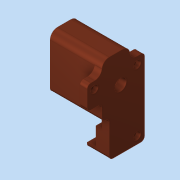
# Autodesk Inventor part: limitSwitchPushHolder1
Saved by Autodesk Inventor 2017 (Build 210142000, 142)
## iProperties
Created: 2016-12-04
Part Number: limitSwitchPushHolder1
Material: ABS Plastic
Document SubType Name: Modeling
Designer: techn
Density: 1.06 g/cm^3
Appearance: Copper - Satin
Author: techn
Autodesk Inventor part; units mm, degrees
ref_plane "YZ Plane" through (0, 0, 0) normal (1, 0, 0) x (0, 1, 0)
ref_plane "XZ Plane" through (0, 0, 0) normal (0, 1, 0) x (-1, 0, 0)
ref_plane "XY Plane" through (0, 0, 0) normal (0, 0, 1) x (1, 0, 0)
sketch "Sketch1" plane through (0, 0, 0) normal (0, 0, 1) x (1, 0, 0)
  line L0 (0, 0) -> (-2.54, 0)
  line L1 (-2.54, 0) -> (-2.54, 7.62)
  line L2 (-2.54, 7.62) -> (0, 7.62)
  line L3 (0, 7.62) -> (0, 0)
  line L4 (-2.54, 7.62) -> (18.796, 7.62)
  line L5 (18.796, 7.62) -> (18.796, 10.16)
  line L6 (18.796, 10.16) -> (-2.54, 10.16)
  line L7 (-2.54, 10.16) -> (-2.54, 7.62)
  line L8 (11.43, -20.32) -> (16.256, -20.32)
  line L9 (16.256, -20.32) -> (16.256, -22.86)
  line L10 (16.256, -22.86) -> (11.43, -22.86)
  line L11 (11.43, -22.86) -> (11.43, -20.32)
  line L12 (16.256, -22.86) -> (18.796, -22.86)
  line L13 (18.796, -22.86) -> (18.796, -12.7)
  line L14 (18.796, -12.7) -> (16.256, -12.7)
  line L15 (16.256, -12.7) -> (16.256, -22.86)
  line L16 (-2.54, 10.16) -> (18.796, 10.16)
  line L17 (18.796, 10.16) -> (18.796, -22.86)
  line L18 (18.796, -22.86) -> (-2.54, -22.86)
  line L19 (-2.54, -22.86) -> (-2.54, 10.16)
  dimension "d0" = 2.54
  dimension "d1" = 7.62
  dimension "d3" = 2.54
  dimension "d4" = 27.94
  dimension "d5" = 11.43
  dimension "d6" = 4.826
  dimension "d7" = 2.54
  dimension "d8" = 2.54
  dimension "d9" = 10.16
  constraints: 40 end point, 10 parallel, 5 horizontal, 5 perpendicular, 1 point on line
  measures "d0" distance of L1.end L2.end
  measures "d1" distance of L0.end L1.end
  measures "d3" distance of L5.end L4.end
  measures "d4" distance from line of L8.start L4
  measures "d5" horizontal distance of L2.end L8.start
  measures "d6" distance of L9.end L10.end
  measures "d7" distance of L8.end L9.end
  measures "d8" distance of L14.end L13.end
  measures "d9" distance of L13.end L12.end
extrude "Extrusion1" add sketch "Sketch1" against normal blind 8.89 contours L0 L1 L2 L3 | L2 L7 L6 L5 L4 | L11 L8 L9 L10 | L13 L12 L9 L15 L14
extrude "Extrusion2" add sketch "Sketch1" along normal blind 3.175
sketch "Sketch5" plane through (18.796, -22.86, -8.89) normal (1, 0, 0) x (0, 0, -1)
  line L0 (-8.89, 33.02) -> (-12.065, 33.02) projected
  line L1 (-12.065, 0) -> (0, 0) projected
  line L2 (0, 33.02) -> (0, 30.48) projected
  line L3 (-18.415, 33.02) -> (6.35, 33.02)
  line L4 (6.35, 33.02) -> (6.35, 0)
  line L5 (6.35, 0) -> (-18.415, 0)
  line L6 (-18.415, 0) -> (-18.415, 33.02)
  line L7 (-12.065, 0) -> (-12.065, 33.02) projected
  circle A0 centre (-15.24, 29.845) radius 1.5875
  circle A1 centre (3.175, 29.845) radius 1.5875
  circle A2 centre (-15.24, 3.175) radius 1.5875
  circle A3 centre (3.175, 3.175) radius 1.5875
  point P0 (-8.89, 22.86)
  dimension "d27" = 6.35
  dimension "d28" = 6.35
  dimension "d29" = 3.175
  dimension "d30" = 3.175
  dimension "d31" = 3.175
  dimension "d32" = 3.175
  dimension "d33" = 3.175
  dimension "d34" = 3.175
  dimension "d35" = 3.175
  dimension "d36" = 3.175
  dimension "d37" = 3.175
  dimension "d38" = 3.175
  dimension "d39" = 3.175
  dimension "d40" = 3.175
  constraints: 8 end point, 4 centre point, 2 parallel, 1 horizontal, 1 perpendicular
  measures "d27" distance between parallel lines of L7 L6
  measures "d28" distance between parallel lines of L2 L4
  measures "d29" diameter of A0
  measures "d30" diameter of A1
  measures "d31" diameter of A2
  measures "d32" diameter of A3
  measures "d33" distance from line of L7 A0.centre
  measures "d34" distance from line of A1.centre L2
  measures "d35" distance from line of L2 A3.centre
  measures "d36" distance from line of L7 A2.centre
  measures "d37" distance from line of L5 A2.centre
  measures "d38" distance from line of L3 A0.centre
  measures "d39" distance from line of L3 A1.centre
  measures "d40" distance from line of L5 A3.centre
extrude "Extrusion5" add sketch "Sketch5" along normal blind 3.175
chamfer "Chamfer2" distance 1.27 angle 45 4 edges at (18.796, 6.985, -10.4775) (18.796, -19.685, -10.4775) (18.796, -19.685, 7.9375) (18.796, 6.985, 7.9375)
sketch "Sketch7" plane through (21.971, -22.86, -8.89) normal (1, 0, 0) x (0, 0, -1)
  line L0 (-8.89, 10.16) -> (-8.89, 30.48) projected
  circle A0 centre (-4.0005, 25.908) radius 2.54
  line L1 (6.35, 33.02) -> (-18.415, 33.02) projected
  point P0 (-8.89, 22.86)
  dimension "d52" = 5.08
  dimension "d53" = 4.8895
  dimension "d54" = 7.112
  constraints: 1 centre point
  measures "d52" diameter of A0
  measures "d53" distance from line of A0.centre L0
  measures "d54" distance from line of A0.centre L1
extrude "Extrusion7" cut sketch "Sketch7" against normal blind 3.175
sketch "Sketch9" plane through (21.971, -22.86, -8.89) normal (1, 0, 0) x (0, 0, -1)
  line L0 (-18.415, 33.02) -> (-18.415, 0) projected
  line L1 (6.35, 33.02) -> (-18.415, 33.02) projected
  line L2 (-18.415, 0) -> (6.35, 0) projected
  line L3 (-18.415, 22.86) -> (-12.065, 22.86)
  line L4 (-12.065, 22.86) -> (-12.065, 0)
  line L5 (-12.065, 0) -> (-18.415, 0)
  line L6 (-18.415, 0) -> (-18.415, 22.86)
  point P0 (-8.89, 22.86)
  dimension "d59" = 6.35
  dimension "d60" = 22.86
  constraints: 8 end point, 2 parallel, 2 point on line, 1 horizontal, 1 perpendicular
  measures "d59" distance of L4.end L5.end
  measures "d60" distance of L3.end L4.end
extrude "Extrusion8" cut sketch "Sketch9" against normal through all
sketch "Sketch12" plane through (0, 0, -8.89) normal (0, 0, -1) x (-1, 0, 0)
  line L0 (-11.43, -20.32) -> (-11.43, -22.86) projected
  line L1 (2.54, -22.86) -> (-21.971, -22.86) projected
  line L2 (-11.43, -20.32) -> (-12.446, -20.32)
  line L3 (-12.446, -20.32) -> (-12.446, -22.86)
  line L4 (-12.446, -22.86) -> (-11.43, -22.86)
  line L5 (-11.43, -22.86) -> (-11.43, -20.32)
  point P0 (0, 0)
  dimension "d69" = 1.016
  constraints: 8 end point, 2 parallel, 1 horizontal, 1 perpendicular, 1 point on line
  measures "d69" distance of L4.end L3.end
extrude "Extrusion9" cut sketch "Sketch12" against normal up to surface (8.89 mm away)
sketch "Sketch16" plane through (21.971, -22.86, -8.89) normal (1, 0, 0) x (0, 0, -1)
  line L0 (-8.89, 10.16) -> (-8.89, 30.48) projected
  line L1 (-12.065, 33.02) -> (-12.065, 0) projected
  line L2 (-8.89, 22.86) -> (-8.89, 0) projected
  line L3 (-12.065, 15.875) -> (-8.89, 15.875)
  line L4 (-8.89, 15.875) -> (-8.89, 0)
  line L5 (-8.89, 0) -> (-12.065, 0)
  line L6 (-12.065, 0) -> (-12.065, 15.875)
  dimension "d74" = 15.875
  constraints: 8 end point, 2 parallel, 1 horizontal, 1 perpendicular, 1 point on line
  measures "d74" distance between parallel lines of L5 L3
extrude "Extrusion10" cut sketch "Sketch16" against normal through all
fillet "Fillet1" radius 1.5875 2 edges at (9.7155, -6.985, 3.175) (20.3835, -6.985, 0)
fillet "Fillet2" radius 1.5875 6 edges at (20.3835, 0, 9.525) (20.3835, 0, 3.175) (17.2085, -22.86, 0) (20.3835, -22.86, -15.24) (20.3835, 10.16, -15.24) (20.3835, 10.16, 9.525)
sketch "Sketch17" plane through (-2.54, 0, -8.89) normal (-1, 0, 0) x (0, 0, 1)
  arc A0 (10.4775, -6.985) -> (12.065, -5.3975) centre (10.4775, -5.3975) ccw projected
  line L0 (12.065, 10.16) -> (12.065, -5.3975) projected
  line L1 (0, 10.16) -> (12.065, 10.16) projected
  line L2 (0, 0) -> (0, 10.16) projected
  line L3 (8.89, 0) -> (0, 0) projected
  line L4 (8.89, 0) -> (8.89, -6.985) projected
  line L5 (8.89, -6.985) -> (10.4775, -6.985) projected
  line L6 (8.89, 7.62) -> (0, 7.62) projected
  line L7 (0, 0) -> (8.89, 0)
  line L8 (8.89, 0) -> (8.89, 7.62)
  line L9 (8.89, 7.62) -> (0, 7.62)
  line L10 (0, 7.62) -> (0, 0)
  constraints: 8 end point, 2 parallel, 1 horizontal, 1 perpendicular
extrude "Extrusion11" cut sketch "Sketch17" against normal up to surface (2.54 mm away) contours L3 L2 L6 L8
sketch "Sketch18" plane through (12.446, -20.32, -8.89) normal (0, 1, 0) x (1, 0, 0)
  line L0 (0, 0) -> (0, -8.89) projected
  line L1 (3.81, -8.89) -> (0, -8.89) projected
  line L2 (3.81, -8.89) -> (3.81, 0) projected
  line L3 (0, 0) -> (3.81, 0) projected
  point P0 (-12.446, -8.89)
extrude "Extrusion12" cut sketch "Sketch18" against normal blind 0.508
sketch "Sketch19" plane through (21.971, -22.86, -8.89) normal (1, 0, 0) x (0, 0, -1)
  line L0 (0, 33.02) -> (-12.065, 33.02) projected
  line L1 (0, 33.02) -> (-12.065, 33.02)
  line L2 (-12.065, 33.02) -> (-12.065, 38.735)
  line L3 (-12.065, 38.735) -> (0, 38.735)
  line L4 (0, 38.735) -> (0, 33.02)
  point P0 (-8.89, 22.86)
  dimension "d84" = 5.715
  constraints: 8 end point, 2 parallel, 1 horizontal, 1 perpendicular
  measures "d84" distance of L1.end L2.end
extrude "Extrusion13" add sketch "Sketch19" against normal up to surface (24.511 mm away)
sketch "Sketch20" plane through (-2.54, 7.62, -8.89) normal (-1, 0, 0) x (0, 0, 1)
  line L0 (0, 0) -> (8.89, 0) projected
  line L1 (8.89, 0) -> (8.89, -14.605) projected
  line L2 (8.89, -14.605) -> (10.4775, -14.605) projected
  arc A0 (10.4775, -14.605) -> (12.065, -13.0175) centre (10.4775, -13.0175) ccw projected
  line L3 (12.065, 8.255) -> (12.065, -13.0175) projected
  line L4 (0, 8.255) -> (12.065, 8.255) projected
  line L5 (0, 0) -> (0, 8.255) projected
  point P0 (8.89, -7.62)
extrude "Extrusion14" cut sketch "Sketch20" against normal blind 2.159
sketch "Sketch21" plane through (-0.381, 7.62, -8.89) normal (-1, 0, 0) x (0, 0, 1)
  line L0 (8.89, 0) -> (0, 0) projected
  line L1 (8.89, -14.605) -> (8.89, 0) projected
  line L2 (10.4775, -14.605) -> (8.89, -14.605) projected
  arc A0 (10.4775, -14.605) -> (12.065, -13.0175) centre (10.4775, -13.0175) ccw projected
  line L3 (12.065, 8.255) -> (12.065, -13.0175) projected
  line L4 (0, 8.255) -> (12.065, 8.255) projected
  line L5 (0, 0) -> (0, 8.255) projected
  circle A1 centre (4.445, 4.1275) radius 1.27
  point P0 (8.89, -7.62)
  dimension "d89" = 2.54
  constraints: 1 centre point
  measures "d89" diameter of A1
extrude "Extrusion15" cut sketch "Sketch21" against normal blind 6.35 contours A1
fillet "Fillet4" radius 3.175 4 edges at (10.795, 15.875, -8.89) (10.795, 15.875, 3.175) (20.3835, 10.16, -8.89) (20.3835, 10.16, 3.175)
sketch "Sketch22" plane through (18.796, -22.86, -8.89) normal (-1, 0, 0) x (0, 0, 1)
  line L0 (8.89, 10.16) -> (8.89, 2.032) projected
  line L1 (8.89, 10.16) -> (0, 10.16) projected
  line L2 (0, 2.032) -> (0, 10.16) projected
  line L3 (0, 2.032) -> (8.89, 2.032) projected
  circle A0 centre (4.445, 34.6075) radius 1.27 projected
  arc A1 (12.065, 35.56) -> (8.89, 38.735) centre (8.89, 35.56) ccw projected
  line L4 (3.175, 38.735) -> (8.89, 38.735) projected
  arc A2 (3.175, 38.735) -> (0, 35.56) centre (3.175, 35.56) ccw projected
  line L5 (0, 30.48) -> (0, 35.56) projected
  line L6 (8.89, 30.48) -> (0, 30.48) projected
  line L7 (8.89, 15.875) -> (8.89, 30.48) projected
  line L8 (10.4775, 15.875) -> (8.89, 15.875) projected
  arc A3 (10.4775, 15.875) -> (12.065, 17.4625) centre (10.4775, 17.4625) ccw projected
  line L9 (12.065, 35.56) -> (12.065, 17.4625) projected
  line L10 (-1.5875, 16.51) -> (-6.0325, 16.51)
  line L11 (-6.0325, 16.51) -> (-6.0325, 24.13)
  line L12 (-6.0325, 24.13) -> (-1.5875, 24.13)
  line L13 (-1.5875, 24.13) -> (-1.5875, 16.51)
  point P0 (8.89, 22.86)
  dimension "d93" = 6.35
  dimension "d94" = 6.35
  dimension "d95" = 1.5875
  dimension "d96" = 4.445
  constraints: 8 end point, 2 parallel, 1 horizontal, 1 perpendicular
  measures "d93" distance between parallel lines of L12 L6
  measures "d94" distance between parallel lines of L10 L1
  measures "d95" distance between parallel lines of L5 L13
  measures "d96" distance of L10.start L10.end
extrude "Extrusion16" add sketch "Sketch22" along normal up to surface (19.177 mm away) contours L10 L11 L12 L13
fillet "Fillet5" radius 1.27 4 edges at (9.2075, -6.35, -14.9225) (9.2075, -6.35, -10.4775) (9.2075, 1.27, -10.4775) (9.2075, 1.27, -14.9225)
fillet "Fillet6" radius 1.27 8 edges at (18.796, -5.978, -14.5505) (18.796, -2.54, -14.9225) (18.796, 0.898, -14.5505) (18.796, 1.27, -12.7) (18.796, 0.898, -10.8495) (18.796, -2.54, -10.4775) (18.796, -5.978, -10.8495) (18.796, -6.35, -12.7)
equation "\"d30\" = d29"
equation "\"d31\" = d29"
equation "\"d32\" = d29"
body "Solid1"
